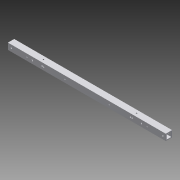
# Autodesk Inventor part: 1x1 horizontal
Saved by Autodesk Inventor 2015 SP1 (Build 190203100, 203)
## iProperties
Created: 2015-01-27
Part Number: 1x1 horizontal
Material: Aluminum 6061
Document SubType Name: Modeling
Designer: Admin
Density: 2.7 g/cm^3
Appearance: Aluminum - Flat
Author: Admin
Autodesk Inventor part; units mm, degrees
ref_plane "YZ Plane" through (0, 0, 0) normal (1, 0, 0) x (0, 1, 0)
ref_plane "XZ Plane" through (0, 0, 0) normal (0, 1, 0) x (-1, 0, 0)
ref_plane "XY Plane" through (0, 0, 0) normal (0, 0, 1) x (1, 0, 0)
sketch "Sketch1" plane through (0, 0, 0) normal (1, 0, 0) x (0, 1, 0)
  line L0 (0, 0) -> (25.4, 0)
  line L1 (25.4, 0) -> (25.4, -25.4)
  line L2 (25.4, -25.4) -> (0, -25.4)
  line L3 (0, -25.4) -> (0, 0)
  line L4 (3.175, -3.175) -> (22.225, -3.175)
  line L5 (22.225, -3.175) -> (22.225, -22.225)
  line L6 (22.225, -22.225) -> (3.175, -22.225)
  line L7 (3.175, -22.225) -> (3.175, -3.175)
  dimension "d0" = 25.4
  dimension "d1" = 25.4
  dimension "d2" = 19.05
  dimension "d3" = 19.05
  dimension "d4" = 3.175
  dimension "d5" = 3.175
  constraints: 16 end point, 4 parallel, 2 horizontal, 2 perpendicular
  measures "d0" distance of L1.end L2.end
  measures "d1" distance of L0.end L1.end
  measures "d2" distance of L5.end L6.end
  measures "d3" distance of L4.end L5.end
  measures "d4" distance between parallel lines of L0 L4
  measures "d5" distance between parallel lines of L3 L7
extrude "Extrusion1" add sketch "Sketch1" along normal blind 635
sketch "Sketch2" plane through (0, 0, 0) normal (0, 0, 1) x (1, 0, 0)
  line L0 (0, 0) -> (0, 25.4) projected
  line L1 (0, 0) -> (635, 0) projected
  line L2 (635, 25.4) -> (635, 0) projected
  point P0 (536.575, 12.7)
  point P1 (498.475, 12.7)
  point P2 (136.525, 12.7)
  point P3 (98.425, 12.7)
  dimension "d8" = 98.425
  dimension "d9" = 38.1
  dimension "d10" = 12.7
  dimension "d11" = 12.7
  dimension "d12" = 12.7
  dimension "d13" = 98.425
  dimension "d14" = 38.1
  dimension "d15" = 12.7
  measures "d8" distance from line of L0 point (98.425, 12.7)
  measures "d9" distance of point (98.425, 12.7) point (136.525, 12.7)
  measures "d10" distance from line of L1 point (98.425, 12.7)
  measures "d11" distance from line of L1 point (136.525, 12.7)
  measures "d12" distance from line of L1 point (536.575, 12.7)
  measures "d13" distance from line of L2 point (536.575, 12.7)
  measures "d14" distance of point (536.575, 12.7) point (498.475, 12.7)
  measures "d15" distance from line of L1 point (498.475, 12.7)
hole "Hole1" at (536.575, 12.7, 0) at (498.475, 12.7, 0) at (136.525, 12.7, 0) at (98.425, 12.7, 0) direction (0, 0, -1) diameter 6.35 end through all
sketch "Sketch3" plane through (0, 0, 0) normal (0, 0, 1) x (1, 0, 0)
  line L0 (0, 0) -> (0, 25.4) projected
  line L1 (0, 0) -> (635, 0) projected
  line L2 (635, 25.4) -> (635, 0) projected
  point P0 (12.7, 12.7)
  point P1 (622.3, 12.7)
  dimension "d23" = 12.7
  dimension "d24" = 12.7
  dimension "d25" = 12.7
  dimension "d26" = 12.7
  measures "d23" distance from line of L1 point (12.7, 12.7)
  measures "d24" distance from line of L0 point (12.7, 12.7)
  measures "d25" distance from line of L2 point (622.3, 12.7)
  measures "d26" distance from line of L1 point (622.3, 12.7)
hole "Hole2" at (12.7, 12.7, 0) at (622.3, 12.7, 0) direction (0, 0, -1) diameter 6.35 end through all
sketch "Sketch4" plane through (0, 0, 0) normal (0, 0, 1) x (1, 0, 0)
  line L0 (0, 0) -> (0, 25.4) projected
  line L1 (0, 0) -> (635, 0) projected
  line L2 (635, 25.4) -> (635, 0) projected
  point P0 (76.2, 12.7)
  point P1 (228.6, 12.7)
  point P2 (406.4, 12.7)
  point P3 (558.8, 12.7)
  dimension "d34" = 12.7
  dimension "d35" = 12.7
  dimension "d36" = 12.7
  dimension "d37" = 12.7
  dimension "d38" = 76.2
  dimension "d39" = 228.6
  dimension "d40" = 228.6
  dimension "d41" = 76.2
  measures "d34" distance from line of L1 point (76.2, 12.7)
  measures "d35" distance from line of L1 point (228.6, 12.7)
  measures "d36" distance from line of L1 point (406.4, 12.7)
  measures "d37" distance from line of L1 point (558.8, 12.7)
  measures "d38" distance from line of L0 point (76.2, 12.7)
  measures "d39" distance from line of L0 point (228.6, 12.7)
  measures "d40" distance from line of L2 point (406.4, 12.7)
  measures "d41" distance from line of L2 point (558.8, 12.7)
hole "Hole3" at (76.2, 12.7, 0) at (228.6, 12.7, 0) at (406.4, 12.7, 0) at (558.8, 12.7, 0) direction (0, 0, -1) diameter 4.7625 end through all
sketch "Sketch6" plane through (0, 0, -25.4) normal (0, 0, -1) x (-1, 0, 0)
  circle A0 centre (-136.525, 12.7) radius 3.175 projected
  circle A1 centre (-498.475, 12.7) radius 3.175 projected
  line L0 (0, 0) -> (-635, 0) projected
  circle A2 centre (-492.125, 12.7) radius 3.175
  circle A3 centre (-142.875, 12.7) radius 3.175
  dimension "d61" = 6.35
  dimension "d62" = 6.35
  dimension "d63" = 6.35
  dimension "d64" = 12.7
  dimension "d65" = 6.35
  dimension "d66" = 12.7
  constraints: 2 centre point
  measures "d61" diameter of A2
  measures "d62" diameter of A3
  measures "d63" distance of A1.centre A2.centre
  measures "d64" distance from line of L0 A2.centre
  measures "d65" distance of A0.centre A3.centre
  measures "d66" distance from line of L0 A3.centre
extrude "Extrusion2" cut sketch "Sketch6" against normal blind 25.4 contours A3 | A2
sketch "Sketch7" plane through (0, 25.4, 0) normal (0, 1, 0) x (1, 0, 0)
  line L0 (635, 25.4) -> (635, 0) projected
  line L1 (0, 25.4) -> (635, 25.4) projected
  point P0 (504.825, 12.7)
  point P1 (130.175, 12.7)
  dimension "d69" = 12.7
  dimension "d70" = 130.175
  dimension "d71" = 12.7
  dimension "d81" = 374.65
  measures "d69" distance from line of L1 point (504.825, 12.7)
  measures "d70" distance from line of L0 point (504.825, 12.7)
  measures "d71" distance from line of L1 point (130.175, 12.7)
  measures "d81" distance of point (504.825, 12.7) point (130.175, 12.7)
hole "Hole5" at (504.825, 25.4, -12.7) at (130.175, 25.4, -12.7) direction (0, -1, 0) diameter 4.7625 depth 25.4 tip angle 118
body "Solid1"
